servo_mount_house (Autodesk Fusion 360 design; units mm, degrees)
Autodesk Fusion 360 part; units mm, degrees
sketch "Sketch1" plane through (0, 0, 0) normal (0, 0, 1) x (1, 0, 0)
  line L0 (0, 0) -> (23.3, 0)
  line L1 (23.3, 0) -> (23.3, 12.5)
  line L2 (23.3, 12.5) -> (0, 12.5)
  line L3 (0, 12.5) -> (0, 0)
  line L4 (0, 6.25) -> (-2.35, 6.25) construction
  line L5 (23.3, 6.25) -> (25.65, 6.25) construction
  circle A0 centre (-2.35, 6.25) radius 1.45
  circle A1 centre (25.65, 6.25) radius 1.45
  line L6 (-4.8, -2) -> (28.1, -2)
  line L7 (28.1, -2) -> (28.1, 12.5)
  line L8 (28.1, 12.5) -> (-4.8, 12.5)
  line L9 (-4.8, 12.5) -> (-4.8, -2)
  dimension "d1" = 23.3
  dimension "d2" = 12.5
  dimension "d3" = 2.35
  dimension "d4" = 2.35
  dimension "d5" = 2.9
  dimension "d6" = 2.9
  dimension "d7" = 2
  dimension "d8" = 2.45
  dimension "d9" = 2.45
  constraint horizontal L0
  constraint vertical L1
  constraint horizontal L2
  constraint vertical L3
  constraint coincident L0.start L3.end
  constraint midpoint L3 L4.start
  constraint perpendicular L3 L4
  constraint midpoint L1 L5.start
  constraint perpendicular L1 L5
  constraint coincident L4.end A0.centre
  constraint coincident L5.end A1.centre
  constraint horizontal L6
  constraint vertical L7
  constraint horizontal L8
  constraint vertical L9
  constraint coincident L2.end L8
  measures "d1" distance of L0.start L0.end
  measures "d2" distance of L0.start L2.end
  measures "d3" distance of L4.start L4.end
  measures "d4" distance of L5.start L5.end
  measures "d5" diameter of A0
  measures "d6" diameter of A1
  measures "d7" distance of L0 L6
  measures "d8" distance of L4.end L9
  measures "d9" distance of L5.end L7
extrude "Extrude1" add sketch "Sketch1" along normal blind 2 contours L0 L1 L3 L6 L7 L8 L9
sketch "Sketch2" plane through (0, 0, 2) normal (0, 0, 1) x (-1, 0, 0)
  circle A0 centre (2.35, -6.25) radius 1.45
  circle A1 centre (-25.65, -6.25) radius 1.45
  line L0 (0, -12.5) -> (4.8, -12.5)
  line L1 (4.8, -12.5) -> (4.8, 2)
  line L2 (4.8, 2) -> (-28.1, 2)
  line L3 (-28.1, 2) -> (-28.1, -12.5)
  line L4 (-28.1, -12.5) -> (-23.3, -12.5)
  line L5 (-23.3, -12.5) -> (-23.3, 0)
  line L6 (-23.3, 0) -> (0, 0)
  line L7 (0, 0) -> (0, -12.5)
